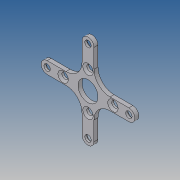
# Autodesk Inventor part: Motorkreuz
Saved by Autodesk Inventor 2019.4 (Build 234330000, 330)
## iProperties
Part Number: Motorkreuz
Material: GEDA Stahl
Document SubType Name: Modeling
Designer: Admin
Mass: 6.29291 g
Surface Area: 13.6412 cm^2
Volume: 0.800624 cm^3
Density: 7.86 g/cm^3
Appearance: GEDA Stahl A
Gewicht: 0,006 kg
G_L: 0
G_H: 0
G_B: 0
InventorVersion: 2019.4
VAULT_Status: in Bearbeitung
Revision: -
Max. Breite: 0
Max. Höhe: 0
Max. Länge: 0
Max. Abmessungen: 0 x 0 x 0
Volumen: 800,624
Author: Admin
Autodesk Inventor part; units mm, degrees
note: some values were not read from the file. Left out: dimensions or parameters whose unit could not be read.
ref_plane "YZ Plane" through (0, 0, 0) normal (1, 0, 0) x (0, 1, 0)
ref_plane "XZ Plane" through (0, 0, 0) normal (0, 1, 0) x (-1, 0, 0)
ref_plane "XY Plane" through (0, 0, 0) normal (0, 0, 1) x (1, 0, 0)
sketch "Skizze1" plane through (0, 0, 0) normal (0, 1, 0) x (-1, 0, 0)
  line L0 (-23.5, -3) -> (23.5, -3)
  line L1 (23.5, -3) -> (23.5, 3)
  line L2 (23.5, 3) -> (-23.5, 3)
  line L3 (-23.5, 3) -> (-23.5, -3)
  line L4 (-23.5, -3) -> (23.5, 3) construction
  line L5 (23.5, -3) -> (-23.5, 3) construction
  line L6 (3, -23.5) -> (-3, -23.5)
  line L7 (-3, -23.5) -> (-3, 23.5)
  line L8 (-3, 23.5) -> (3, 23.5)
  line L9 (3, 23.5) -> (3, -23.5)
  line L10 (3, -23.5) -> (-3, 23.5) construction
  line L11 (-3, -23.5) -> (3, 23.5) construction
  point P0 (0, 0)
  dimension "d0" = 6
  dimension "d1" = 47
  constraints: 24 end point, 4 midpoint, 4 parallel, 4 perpendicular, 2 horizontal
  measures "d0" distance of L7.end L8.end
  measures "d1" distance of L6.end L7.end
extrude "Extrusion1" add sketch "Skizze1" along normal blind 2
sketch "Skizze2" plane through (0, 0, 0) normal (0, -1, 0) x (1, 0, 0)
  circle A0 centre (0, 20.5) radius 1.6
  circle A1 centre (0, -20.5) radius 1.6
  circle A2 centre (20.5, 0) radius 1.6
  circle A3 centre (-20.5, 0) radius 1.6
  line L0 (0, 20.5) -> (0, -20.5) construction
  line L1 (3, -3) -> (3, -23.5) construction
  line L2 (20.5, 0) -> (-20.5, 0) construction
  circle A4 centre (0, 9.5) radius 1.6
  circle A5 centre (0, -9.5) radius 1.6
  circle A6 centre (12.5, 0) radius 1.6
  circle A7 centre (-12.5, 0) radius 1.6
  line L3 (0, 9.5) -> (0, -9.5) construction
  line L4 (12.5, 0) -> (-12.5, 0) construction
  point P0 (0, 0)
  point P1 (0, 0)
  dimension "d4" = 3.2
  dimension "d5" = 41
  dimension "d7" = 19
  dimension "d8" = 25
  constraints: 8 centre point, 8 end point, 7 equal radius, 4 midpoint, 4 point on line, 2 perpendicular, 1 coincident, 1 collinear, 1 horizontal, 1 parallel
  measures "d4" diameter of A0
  measures "d5" distance of L2.start L2.end
  measures "d7" distance of L3.end L3.start
  measures "d8" distance of L4.start L4.end
extrude "Extrusion2" cut sketch "Skizze2" against normal blind 2
fillet "Rundung1" radius 3 8 edges at (-3, 1, 23.5) (3, 1, 23.5) (23.5, 1, 3) (23.5, 1, -3) (3, 1, -23.5) (-3, 1, -23.5) (-23.5, 1, -3) (-23.5, 1, 3)
fillet "Rundung2" radius 8 4 edges at (3, 1, 3) (-3, 1, 3) (-3, 1, -3) (3, 1, -3)
sketch "Skizze3" plane through (0, 0, 0) normal (0, -1, 0) x (1, 0, 0)
  circle A0 centre (0, 0) radius 5
  dimension "d13" = 10
  constraints: 1 centre point, 1 coincident
  measures "d13" diameter of A0
extrude "Extrusion3" cut sketch "Skizze3" against normal blind 2
chamfer "Fase1" distance 1 angle 45 8 edges at (-1.6, 0, 9.5) (-14.1, 0, 0) (10.9, 0, 0) (-1.6, 0, -9.5) (-1.6, 2, 20.5) (-22.1, 2, 0) (18.9, 2, 0) (-1.6, 2, -20.5)
equation "\"G_L\" = 0"
equation "\"G_H\" = 0"
equation "\"G_B\" = 0"
